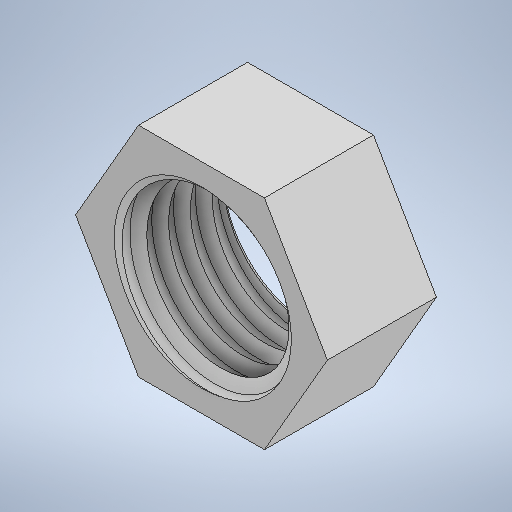
# Autodesk Inventor part: Nut 1.1
Saved by Autodesk Inventor 2025.2 (Build 292293000, 293)
## iProperties
Created: 2024-11-18
Part Number: Nut 1.1
Material: Generic
Document SubType Name: Modeling
Designer: jurre
Density: 1 g/cm^3
Appearance: Default
Author: jurre
Autodesk Inventor part; units mm, degrees
ref_plane "YZ Plane" through (0, 0, 0) normal (1, 0, 0) x (0, 1, 0)
ref_plane "XZ Plane" through (0, 0, 0) normal (0, 1, 0) x (-1, 0, 0)
ref_plane "XY Plane" through (0, 0, 0) normal (0, 0, 1) x (1, 0, 0)
sketch "Sketch1" plane through (0, 0, 0) normal (0, 0, 1) x (1, 0, 0)
  line L0 (2.8868, 5) -> (5.7735, 0)
  line L1 (5.7735, 0) -> (2.8868, -5)
  line L2 (2.8868, -5) -> (-2.8868, -5)
  line L3 (-2.8868, -5) -> (-5.7735, 0)
  line L4 (-5.7735, 0) -> (-2.8868, 5)
  line L5 (-2.8868, 5) -> (2.8868, 5)
  point P0 (0, 0)
  point P1 (0, 0)
  dimension "d0" = 10
  constraints: 12 end point, 1 coincident, 13 other
  measures "d0" distance between parallel lines of L2 L5
extrude "Extrusion1" add sketch "Sketch1" along normal blind 5
sketch "Sketch2" plane through (0, 0, 5) normal (0, 0, 1) x (1, 0, 0)
  circle A0 centre (0, 0) radius 3.5
  dimension "d3" = 7
  constraints: 1 centre point, 1 coincident
  measures "d3" diameter of A0
extrude "Extrusion2" cut sketch "Sketch2" against normal blind 5
chamfer "Chamfer1" distance 0.5 angle 45 1 edges at (-3.5, 0, 5)
chamfer "Chamfer2" distance 0.5 angle 45 1 edges at (-3.5, 0, 0)
sketch "Sketch3" plane through (0, 0, 0) normal (0, 1, 0) x (-1, 0, 0)
  line L0 (-3.5, -0.5) -> (-3.5, -1.5)
  line L1 (-3.5, -1.5) -> (-3.991, -1.2165)
  line L2 (-3.991, -0.7835) -> (-3.5, -0.5)
  line L3 (-3.5, -1) -> (-4.366, -1) construction
  line L4 (-5.7735, 0) -> (-2.8868, 0) projected
  arc A0 (-3.991, -0.7835) -> (-3.991, -1.2165) centre (-3.866, -1) ccw
  line L5 (0, 0) -> (0, -5.6606)
  dimension "d14" = 0.5
  dimension "d16" = 60
  dimension "d17" = 1
  dimension "d18" = 0.25
  dimension "d19" = 3.5
  constraints: 10 end point, 2 point on circle, 2 point on line, 2 tangent, 2 vertical, 1 centre point, 1 midpoint, 1 perpendicular
  measures "d14" distance from line of L4 L0.start
  measures "d16" angle of L2 L1
  measures "d17" distance of L0.start L0.end
  measures "d18" radius of A0
  measures "d19" distance from line of L5 L3.start
coil "Coil1" sketch "Sketch3" operation cut axis through (0, 0, -10) along (0, 0, 1) pitch 1 turns 7 hand right
body "Solid1"
